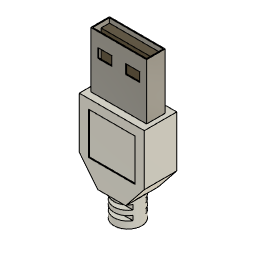
反应堆接口 v1 v1 (Autodesk Fusion 360 design; units mm, degrees)
Autodesk Fusion 360 part; units mm, degrees
note: some values were not read from the file. Set by a fixed rule: which sketch regions a step uses.
sketch "草图1" plane through (0, 0, 0) normal (0, 1, 0) x (1, 0, 0)
  line L0 (0, 0) -> (14, 0)
  line L1 (14, 0) -> (14, -11)
  line L2 (14, -11) -> (0, -11)
  line L3 (0, -11) -> (0, 0)
  line L4 (7, -11) -> (7, 8) construction
  line L5 (7, 5) -> (10, 5)
  line L6 (7, 5) -> (4, 5)
  line L7 (0, 0) -> (4, 5)
  line L8 (14, 0) -> (10, 5)
  dimension "d1" = 14
  dimension "d2" = 11
  dimension "d3" = 3
  dimension "d4" = 3
  dimension "d5" = 5
  constraint horizontal L0
  constraint vertical L1
  constraint horizontal L2
  constraint vertical L3
  constraint coincident L0.start L3.end
  constraint midpoint L2 L4.start
  constraint perpendicular L0 L4
  constraint coincident L4 L5.start
  constraint perpendicular L4 L5
  constraint perpendicular L4 L6
  measures "d1" distance of L0.start L0.end
  measures "d2" distance of L0.start L2.end
  measures "d3" distance of L5.start L5.end
  measures "d4" distance of L5.start L6.end
  measures "d5" distance of L0 L6
extrude "拉伸1" add sketch "草图1" along normal blind 7
sketch "草图2" plane through (0, 0, 11) normal (0, 0, 1) x (-1, 0, 0)
  line L0 (0, 0) -> (-14, 0)
  line L1 (-14, 0) -> (-14, -7)
  line L2 (-14, -7) -> (0, -7)
  line L3 (0, -7) -> (0, 0)
  line L4 (-1, -5.5) -> (-13, -5.5)
  line L5 (-13, -5.5) -> (-13, -1.5)
  line L6 (-13, -1.5) -> (-1, -1.5)
  line L7 (-1, -1.5) -> (-1, -5.5)
  line L8 (-1.2, -1.7) -> (-1.2, -5.3)
  line L9 (-1.2, -5.3) -> (-12.8, -5.3)
  line L10 (-12.8, -5.3) -> (-12.8, -1.7)
  line L11 (-12.8, -1.7) -> (-1.2, -1.7)
  line L12 (-1.2, -3.5) -> (-12.8, -3.5)
  dimension "d8" = 12
  dimension "d9" = 4
  dimension "d10" = 1.5
  dimension "d11" = 1
  dimension "d12" = 0.2
  constraint horizontal L4
  constraint vertical L5
  constraint horizontal L6
  constraint vertical L7
  constraint midpoint L8 L12.start
  constraint midpoint L10 L12.end
  measures "d8" distance of L4.start L4.end
  measures "d9" distance of L4.start L6.end
  measures "d10" distance of L2 L4
  measures "d11" distance of L3 L7
extrude "拉伸2" add sketch "草图2" along normal blind 12 contours L4 L5 L6 L7
extrude "拉伸3" add sketch "草图2" along normal blind 11 contours L8 L9 L10 L12
sketch "草图3" plane through (0, 0, 0) normal (0, -1, 0) x (1, 0, 0)
  line L0 (14, 0) -> (14, 11)
  line L1 (14, 11) -> (0, 11)
  line L2 (0, 11) -> (0, 0)
  line L3 (0, 0) -> (4, -5)
  line L4 (4, -5) -> (10, -5)
  line L5 (10, -5) -> (14, 0)
  line L6 (2, 9) -> (12, 9)
  line L7 (12, 9) -> (12, 0)
  line L8 (12, 0) -> (2, 0)
  line L9 (2, 0) -> (2, 9)
  constraint horizontal L6
  constraint vertical L7
  constraint horizontal L8
  constraint vertical L9
extrude "拉伸4" cut sketch "草图3" against normal blind 0.2 contours L6 L7 L8 L9
sketch "草图4" plane through (0, 7, 0) normal (0, 1, 0) x (-1, 0, 0)
  line L0 (-14, 11) -> (-14, 0)
  line L1 (-14, 0) -> (-10, -5)
  line L2 (-10, -5) -> (-4, -5)
  line L3 (-4, -5) -> (0, 0)
  line L4 (0, 0) -> (0, 11)
  line L5 (0, 11) -> (-14, 11)
  line L6 (-12, 9) -> (-2, 9)
  line L7 (-2, 9) -> (-2, 0)
  line L8 (-2, 0) -> (-12, 0)
  line L9 (-12, 0) -> (-12, 9)
  constraint horizontal L6
  constraint vertical L7
  constraint horizontal L8
  constraint vertical L9
extrude "拉伸5" cut sketch "草图4" against normal blind 0.2 contours L6 L7 L8 L9
sketch "草图5" plane through (0, 1.5, 0) normal (0, -1, 0) x (1, 0, 0)
  line L0 (1, 11) -> (13, 11)
  line L1 (13, 11) -> (13, 23)
  line L2 (13, 23) -> (1, 23)
  line L3 (1, 23) -> (1, 11)
  line L4 (7, 11) -> (7, 23) construction
  line L5 (2.5, 20) -> (5.5, 20)
  line L6 (5.5, 20) -> (5.5, 18)
  line L7 (5.5, 18) -> (2.5, 18)
  line L8 (2.5, 18) -> (2.5, 20)
  line L9 (11.5, 20) -> (8.5, 20)
  line L10 (11.5, 18) -> (11.5, 20)
  line L11 (8.5, 18) -> (11.5, 18)
  line L12 (8.5, 20) -> (8.5, 18)
  dimension "d21" = 1.5
  constraint midpoint L0 L4.start
  constraint midpoint L2 L4.end
  constraint horizontal L5
  constraint vertical L6
  constraint horizontal L7
  constraint vertical L8
  constraint symmetric L4 L5.start L9.start
  constraint symmetric L4 L5.end L9.end
  constraint symmetric L4 L6.end L11.start
  constraint symmetric L4 L7.end L10.start
  measures "d21" distance of L3 L8
extrude "拉伸6" cut sketch "草图5" against normal up to surface (0.2 mm away) contours L5 L6 L7 L8 | L9 L10 L11 L12
sketch "草图6" plane through (0, 0, -5) normal (0, 0, -1) x (1, 0, 0)
  line L0 (10, 0) -> (4, 0)
  line L1 (4, 0) -> (4, -7)
  line L2 (4, -7) -> (10, -7)
  line L3 (10, -7) -> (10, 0)
  circle A0 centre (6.9717, -3.5) radius 3
  dimension "d24" = 6
  measures "d24" diameter of A0
extrude "拉伸7" add sketch "草图6" along normal blind 5.5 contours L1 A0 picked at (7.5942, -2.8884)
sketch "草图7" plane through (0, 0, 0) normal (0, 1, 0) x (1, 0, 0)
  line L0 (4, 6) -> (10, 6)
  line L1 (10, 6) -> (10, 7)
  line L2 (10, 7) -> (4, 7)
  line L3 (4, 7) -> (4, 6)
  line L4 (4, 8) -> (10, 8)
  line L5 (10, 8) -> (10, 9)
  line L6 (10, 9) -> (4, 9)
  line L7 (4, 9) -> (4, 8)
  constraint horizontal L0
  constraint vertical L1
  constraint horizontal L2
  constraint vertical L3
  constraint horizontal L4
  constraint vertical L5
  constraint horizontal L6
  constraint vertical L7
extrude "拉伸8" cut sketch "草图7" along normal blind 2
extrude "拉伸9" cut 2 faces at (6.1056, 2, -6.3333) (6.1056, 2, -8.3333) along direction (0, 1, 0) blind 2 from surface at 2.5
